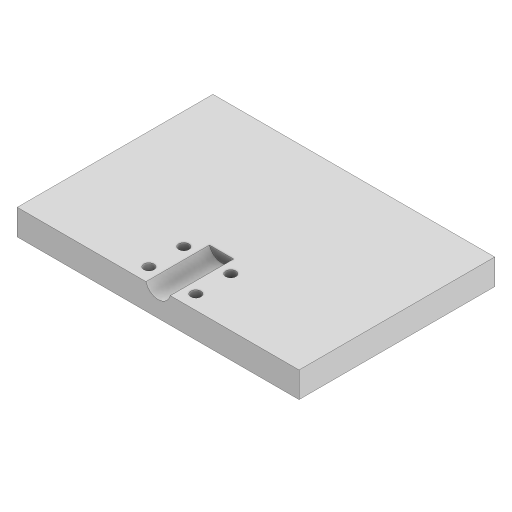
# Autodesk Inventor part: Нижняя часть крепления мотора
Saved by Autodesk Inventor 2023.2 (Build 272271030, 271C)
## iProperties
Created: 2024-12-16
Part Number: Нижняя часть крепления мотора
Material: Типовые
Document SubType Name: Modeling
Designer: I9232
Density: 1 g/cm^3
Appearance: По умолчанию
Author: I9232
Autodesk Inventor part; units mm, degrees
sketch "Эскиз1" plane through (0, 0, 0) normal (0, 1, 0) x (-1, 0, 0)
  line L0 (23.75, 20.25) -> (-23.75, 20.25)
  line L1 (-23.75, 20.25) -> (-23.75, -20.25)
  line L2 (-23.75, -20.25) -> (23.75, -20.25)
  line L3 (23.75, -20.25) -> (23.75, 20.25)
  line L4 (23.75, 20.25) -> (-23.75, -20.25) construction
  circle A0 centre (-15, 11.1546) radius 3.25
  line L5 (-15, 11.1546) -> (-23.75, 11.1546)
  line L6 (-15, 11.1546) -> (-15, 20.25)
  line L7 (-23.75, 20.25) -> (-90, 20.25)
  line L8 (-90, 20.25) -> (-90, -104.75)
  line L9 (0, -7.5) -> (0, 7.5) construction
  line L10 (-126, 0) -> (126, 0) construction
  line L11 (7.5, 0) -> (-7.5, 0) construction
  line L12 (0, -129.75) -> (0, 45.25) projected
  circle A1 centre (15, 11.1546) radius 3.25
  circle A2 centre (-15, -11.1546) radius 3.25
  circle A3 centre (15, -11.1546) radius 3.25
  line L13 (23.75, 20.25) -> (90, 20.25)
  line L14 (90, 20.25) -> (90, -104.75)
  line L15 (90, -104.75) -> (-90, -104.75)
  point P0 (0, 0)
  point P1 (0, 0)
  point P2 (0, 0)
  dimension "d0" = 47.5
  dimension "d1" = 40.5
  dimension "d10" = 8.75
  dimension "d11" = 9.0954
  dimension "d21" = 66.25
  dimension "d22" = 125
  dimension "d23" = 15
  dimension "d24" = 15
  constraints: 28 end point, 6 midpoint, 5 symmetric about line, 4 centre point, 4 perpendicular, 3 horizontal, 3 point on line, 2 parallel, 2 vertical, 3 other
  measures "d0" distance of L1.end L2.end
  measures "d1" distance of L0.end L1.end
  measures "d10" distance of L5.start L5.end
  measures "d11" distance of L5.start L6.end
  measures "d21" distance of L0.end L7.end
  measures "d22" distance of L7.end L8.end
  measures "d23" distance of L9.start L9.end
  measures "d24" distance of L11.start L11.end
extrude "Выдавливание1" add sketch "Эскиз1" along normal blind 16.4 contours L6 A0 L5 L1 L0 | L0 L12 L2 L1 L5 A0 L6 | L1 L2 L12 L15 L8 L7 | L0 L3 L2 L12 | L13 L14 L15 L12 L2 L3
sketch "Эскиз4" plane through (-90, 0, 20.25) normal (0, 0, 1) x (1, 0, 0)
  arc A0 (82.2413, 16.4) -> (97.7587, 16.4) centre (90, 18.35) ccw
  line L0 (0, 16.4) -> (180, 16.4) projected
  line L1 (0, 0) -> (180, 0) projected
  line L2 (66.25, 16.4) -> (113.75, 16.4)
  line L3 (113.75, 16.4) -> (113.75, 0)
  line L4 (113.75, 0) -> (66.25, 0)
  line L5 (66.25, 0) -> (66.25, 16.4)
  line L6 (66.25, 16.4) -> (113.75, 0)
  line L7 (113.75, 16.4) -> (66.25, 0)
  line L8 (90, 22.02) -> (90, -3.67) construction
  point P0 (90, 0)
  point P1 (90, 8.2)
  point P2 (90, 8.2)
  point P3 (97.7587, 16.4)
  dimension "d30" = 16
  dimension "d32" = 47.5
  dimension "d33" = 10.15
  constraints: 12 end point, 6 point on line, 2 midpoint, 2 parallel, 2 point on circle, 1 centre point, 1 horizontal, 1 perpendicular
  measures "d30" diameter of A0
  measures "d32" distance between parallel lines of L3 L5
  measures "d33" distance of point (90, 8.2) A0.centre
extrude "Выдавливание5" cut sketch "Эскиз4" against normal blind 40.5 contours L0 A0
